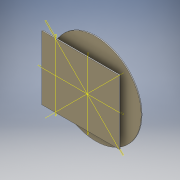
# Autodesk Inventor part: rotating_turntable
Saved by Autodesk Inventor 2016 (Build 200138000, 138)
## iProperties
Created: 2016-01-21
Part Number: rotating_turntable
Material: Generic
Document SubType Name: Modeling
Designer: Fred
Density: 1 g/cm^3
Appearance: Default
Author: Fred
Autodesk Inventor part; units mm, degrees
ref_plane "YZ Plane" through (0, 0, 0) normal (1, 0, 0) x (0, 1, 0)
ref_plane "XZ Plane" through (0, 0, 0) normal (0, 1, 0) x (-1, 0, 0)
ref_plane "XY Plane" through (0, 0, 0) normal (0, 0, 1) x (1, 0, 0)
sketch "Sketch1" plane through (0, 0, 0) normal (0, 1, 0) x (-1, 0, 0)
  line L0 (0, 0) -> (-853.55, 0)
  line L1 (-853.55, 0) -> (-853.55, -707.1)
  line L2 (-853.55, -707.1) -> (0, -707.1)
  line L3 (0, -707.1) -> (0, 0)
  dimension "d0" = 853.55
  dimension "d1" = 707.1
  constraints: 8 end point, 2 parallel, 1 horizontal, 1 perpendicular
  measures "d0" distance of L2.end L1.end
  measures "d1" distance of L1.end L0.end
extrude "Extrusion1" add sketch "Sketch1" along normal blind 10
ref_plane "Work Plane4" through (500, 0, 0) normal (1, 0, 0) x (0, 0, -1)
ref_plane "Work Plane3" through (146.45, 0, 0) normal (1, 0, 0) x (0, 0, -1)
ref_plane "Work Plane2" through (853.55, 0, -353.55) normal (0, 0, -1) x (-1, 0, 0)
ref_plane "Work Plane5" through (500, 0, -353.55) normal (0.7071, 0, -0.7071) x (0, 1, 0)
ref_plane "Work Plane6" through (500, 0, -353.55) normal (0.7071, 0, 0.7071) x (0, -1, 0)
sketch "Sketch2" plane through (0, 10, 0) normal (0, 1, 0) x (1, 0, 0)
  line L0 (500, 848.52) -> (500, -141.42) projected
  line L1 (1009.615, 863.165) -> (-82.84, -229.29) projected
  line L2 (-170.71, 353.55) -> (1024.26, 353.55) projected
  line L3 (0, 0) -> (853.55, 0) projected
  line L4 (853.55, 0) -> (853.55, 707.1) projected
  line L5 (853.55, 707.1) -> (0, 707.1) projected
  line L6 (0, 707.1) -> (0, 0) projected
  circle A0 centre (500, 353.55) radius 37.5
  dimension "d5" = 75
  constraints: 2 point on line, 1 centre point
  measures "d5" diameter of A0
extrude "Extrusion2" add sketch "Sketch2" along normal blind 85 contours A0 L1 L0 | L0 L2 A0 | L2 A0 L0 | L0 A0 L1 | L1 A0 L2 | L1 A0 L2
sketch "Sketch3" plane through (500, 95, -353.55) normal (0, 1, 0) x (1, 0, 0)
  circle A0 centre (0, 0) radius 500
  point P0 (-500, -353.55)
  dimension "d8" = 1000
  constraints: 1 centre point
  measures "d8" diameter of A0
extrude "Extrusion3" add sketch "Sketch3" along normal blind 10
body "Solid1"
